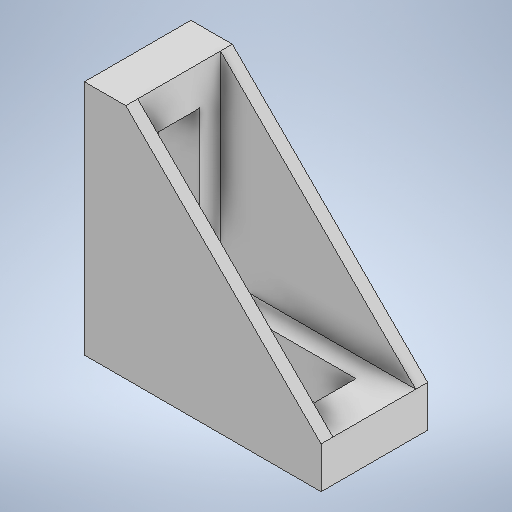
# Autodesk Inventor part: masterpiece_uhelnik
Saved by Autodesk Inventor 2025 (Build 290162000, 162)
## iProperties
Created: 2024-12-16
Part Number: masterpiece_uhelnik
Material: Všeobecné
Document SubType Name: Modeling
Designer: lukas
Density: 1 g/cm^3
Appearance: Výchozí
Author: lukas
## iProperties of the stored document masterpiece_uhelnik_3D tisk.ipt
Created: 2024-12-16
Part Number: masterpiece_uhelnik_3D tisk
Material: Všeobecné
Document SubType Name: Modeling
Designer: lukas
Density: 1 g/cm^3
Appearance: Výchozí
Author: lukas
Autodesk Inventor part; units mm, degrees
ref_plane "YZ Plane" through (0, 0, 0) normal (1, 0, 0) x (0, 1, 0)
ref_plane "XZ Plane" through (0, 0, 0) normal (0, 1, 0) x (-1, 0, 0)
ref_plane "XY Plane" through (0, 0, 0) normal (0, 0, 1) x (1, 0, 0)
sketch "Náčrt1" plane through (0, 0, 0) normal (0, 0, 1) x (1, 0, 0)
  line L0 (-29.3603, 0) -> (36.1619, 0) projected
  line L1 (0, 35.0931) -> (0, -29.1822) projected
  line L2 (-20, -20) -> (20, -20)
  line L3 (20, -20) -> (20, -13)
  line L4 (20, -13) -> (-13, 20)
  line L5 (-13, 20) -> (-20, 20)
  line L6 (-20, 20) -> (-20, -20)
  point P0 (0, 0)
  dimension "d0" = 40
  dimension "d1" = 40
  dimension "d2" = 7
  dimension "d3" = 7
  constraints: 10 end point, 2 perpendicular, 1 horizontal, 1 vertical, 2 other
  measures "d0" distance of L5.end L2.start
  measures "d1" distance of L2.start L2.end
  measures "d2" distance of L2.end L3.end
  measures "d3" distance of L4.end L5.end
extrude "Vysunutí1" add sketch "Náčrt1" along normal blind 18
ref_plane "Pracovní rovina1" through (20, -20, 0) normal (-1, 0, 0) x (0, 0, 1)
sketch "Náčrt2" plane through (20, -20, 0) normal (-1, 0, 0) x (0, 0, 1)
  line L0 (0, -8) -> (0, 48) projected
  line L1 (-3.6, 20) -> (21.6, 20) projected
  line L2 (0, 7) -> (0, 40) projected
  line L3 (0, 40) -> (18, 40) projected
  line L4 (18, 7) -> (18, 40) projected
  line L5 (0, 7) -> (18, 7) projected
  line L6 (2, 7) -> (16, 7)
  line L7 (16, 7) -> (16, 40)
  line L8 (16, 40) -> (2, 40)
  line L9 (2, 40) -> (2, 7)
  point P0 (0, 20)
  point P1 (2, 40)
  dimension "d7" = 14
  dimension "d8" = 2
  constraints: 8 end point, 2 parallel, 2 point on line, 1 horizontal, 1 perpendicular
  measures "d7" distance of L8.end L7.end
  measures "d8" distance between parallel lines of L0 L9
extrude "Vysunutí2" cut sketch "Náčrt2" along normal blind 33 contours L9 L1 L7 L5 | L9 L3 L7 L1
sketch "Náčrt3" plane through (20, -20, 0) normal (-1, 0, 0) x (0, 0, 1)
  line L0 (12.5, 33.4) -> (5.5, 33.4)
  line L1 (5.5, 33.4) -> (5.5, 13)
  line L2 (5.5, 13) -> (12.5, 13)
  line L3 (12.5, 13) -> (12.5, 33.4)
  line L4 (2, 7) -> (16, 7) projected
  line L5 (2, 40) -> (2, 7) projected
  line L6 (2, 40) -> (16, 40) projected
  line L7 (16, 7) -> (16, 40) projected
  line L8 (0, 48) -> (0, -8) projected
  line L9 (-3.6, 20) -> (21.6, 20) projected
  point P0 (0, 20)
  dimension "d11" = 7
  dimension "d12" = 20.4
  dimension "d13" = 6.6
  dimension "d14" = 3.5
  constraints: 8 end point, 2 parallel, 1 horizontal, 1 perpendicular
  measures "d11" distance of L0.start L0.end
  measures "d12" distance of L0.end L1.end
  measures "d13" distance between parallel lines of L0 L6
  measures "d14" distance between parallel lines of L5 L1
extrude "Vysunutí3" cut sketch "Náčrt3" along normal through all contours L3 L9 L1 L0 | L3 L2 L1 L9
ref_plane "Pracovní rovina2" through (-13, 20, 0) normal (0, 1, 0) x (1, 0, 0)
sketch "Náčrt4" plane through (-13, 20, 0) normal (0, 1, 0) x (1, 0, 0)
  line L0 (33, -2) -> (33, -16) projected
  line L1 (33, -2) -> (0, -2) projected
  line L2 (0, -2) -> (0, -16) projected
  line L3 (33, -16) -> (0, -16) projected
  line L4 (13, 3.6) -> (13, -21.6) projected
  line L5 (41, 0) -> (-15, 0) projected
  line L6 (26.4, -5.5) -> (6, -5.5)
  line L7 (6, -5.5) -> (6, -12.5)
  line L8 (6, -12.5) -> (26.4, -12.5)
  line L9 (26.4, -12.5) -> (26.4, -5.5)
  point P0 (13, 0)
  dimension "d17" = 7
  dimension "d18" = 6.6
  dimension "d19" = 20.4
  dimension "d20" = 3.5
  constraints: 8 end point, 2 parallel, 1 horizontal, 1 perpendicular
  measures "d17" distance of L8.end L6.start
  measures "d18" distance between parallel lines of L0 L9
  measures "d19" distance of L6.start L6.end
  measures "d20" distance between parallel lines of L3 L8
extrude "Vysunutí4" cut sketch "Náčrt4" against normal through all contours L6 L9 L8 L4 | L4 L8 L7 L6
